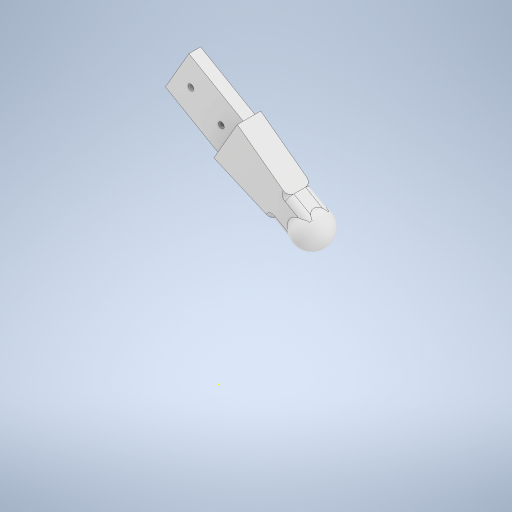
# Autodesk Inventor part: BR_parts_06(2)
Saved by Autodesk Inventor 2024.3 (Build 283343000, 343)
## iProperties
Created: 2024-10-20
Part Number: BR_parts_06(2)
Material: ABS プラスチック
Document SubType Name: Modeling
Designer: 佐藤智貴
Density: 1.06 g/cm^3
Appearance: 滑らか - 白
Mass: 50.0826 g
Surface Area: 111.12 cm^2
Volume: 47.2477 cm^3
Author: 佐藤智貴
Autodesk Inventor part; units mm, degrees
ref_plane "YZ Plane" through (0, 0, 0) normal (1, 0, 0) x (0, 1, 0)
ref_plane "XZ Plane" through (0, 0, 0) normal (0, 1, 0) x (-1, 0, 0)
ref_plane "XY Plane" through (0, 0, 0) normal (0, 0, 1) x (1, 0, 0)
sketch "スケッチ1" plane through (0, 0, 0) normal (0, 0, 1) x (1, 0, 0)
  line L0 (0, 0) -> (40, 0)
  line L1 (40, 0) -> (40, 318)
  line L2 (40, 318) -> (0, 318)
  line L3 (0, 318) -> (0, 0)
  line L4 (0, 218) -> (112.76268, 152.896436)
  line L5 (112.76268, 152.896436) -> (132.76268, 187.537452)
  line L6 (132.76268, 187.537452) -> (40, 241.094011)
  point P0 (40, 218)
  point P1 (40, 194.905989)
  point P2 (20, 318)
  point P3 (122.76268, 170.216944)
  point P4 (20, 258)
  dimension "d0" = 40
  dimension "d1" = 318
  dimension "d69" = 40
  dimension "d70" = 60
  dimension "d91" = 20
  dimension "d92" = 100
  dimension "d93" = 180
  dimension "d96" = 20
  dimension "d97" = 60
  constraints: 14 end point, 3 perpendicular, 3 point on line, 2 midpoint, 2 parallel, 1 horizontal
  measures "d0" distance of L1.end L2.end
  measures "d1" distance of L0.end L1.end
  measures "d69" distance of L4.end L5.end
  measures "d70" angle of L3 L4
  measures "d91" distance from line of L6 point (40, 218)
  measures "d92" distance from line of L2 L4.start
  measures "d93" distance of point (20, 318) point (122.763, 170.217)
  measures "d96" distance from line of L1 point (20, 258)
  measures "d97" distance from line of L2 point (20, 258)
extrude "押し出し1" add sketch "スケッチ1" along normal blind 19.6 contours L3 L2 L1 L4 | L1 L6 L5 L4
sketch "スケッチ6" plane through (0, 0, 19.6) normal (0, 0, 1) x (1, 0, 0)
  circle A0 centre (20, 258) radius 4
  line L0 (40, 318) -> (0, 318)
  line L1 (40, 241.094011) -> (40, 318)
  circle A1 centre (20, 20) radius 1.2295
  circle A2 centre (20, 10) radius 1.2295
  line L2 (0, 0) -> (40, 0)
  circle A3 centre (20, 298) radius 4
  point P0 (20, 318)
  point P1 (40, 190.811367)
  point P2 (30, 0)
  dimension "d42" = 8
  dimension "d44" = 20
  dimension "d45" = 2.459
  dimension "d46" = 2.459
  dimension "d47" = 10
  dimension "d48" = 10
  dimension "d49" = 20
  dimension "d50" = 20
  dimension "d53" = 8
  dimension "d54" = 20
  dimension "d55" = 40
  dimension "d56" = 20
  constraints: 4 centre point, 1 midpoint
  measures "d42" diameter of A0
  measures "d44" distance from line of L1 A0.centre
  measures "d45" diameter of A1
  measures "d46" diameter of A2
  measures "d47" distance from line of L2 A2.centre
  measures "d48" distance of A2.centre A1.centre
  measures "d49" distance from line of L1 A2.centre
  measures "d50" distance from line of L1 A1.centre
  measures "d53" diameter of A3
  measures "d54" distance from line of L0 A3.centre
  measures "d55" distance of A3.centre A0.centre
  measures "d56" distance from line of L1 A3.centre
extrude "押し出し4" cut sketch "スケッチ6" against normal through all
sketch "スケッチ8" plane through (0, 0, 0) normal (-1, 0, 0) x (0, 0, 1)
  line L0 (0, 318) -> (19.6, 318) projected
  line L1 (5, 318) -> (14.6, 318)
  line L2 (14.6, 318) -> (14.6, 278)
  line L3 (14.6, 278) -> (5, 278)
  line L4 (5, 278) -> (5, 318)
  line L5 (0, 318) -> (0, 0) projected
  dimension "d57" = 5
  dimension "d58" = 9.6
  dimension "d59" = 40
  dimension "d98" = 19.6
  constraints: 8 end point, 2 parallel, 1 horizontal, 1 perpendicular, 1 point on line
  measures "d57" distance between parallel lines of L5 L4
  measures "d58" distance between parallel lines of L4 L2
  measures "d59" distance between parallel lines of L0 L3
  measures "d98" distance of L0.start L0.end
extrude "押し出し5" cut sketch "スケッチ8" against normal through all
fillet "フィレット1" radius 20 4 edges at (40, 318, 17.1) (40, 318, 2.5) (0, 318, 2.5) (0, 318, 17.1)
fillet "フィレット2" radius 40 2 edges at (0, 218, 9.8) (40, 241.094, 9.8)
sketch "スケッチ9" plane through (0, 0, 19.6) normal (0, 0, 1) x (1, 0, 0)
  line L0 (20, 206.452995) -> (112.76268, 152.896436)
  line L1 (132.76268, 187.537452) -> (60, 229.547005)
  line L2 (112.76268, 152.896436) -> (132.76268, 187.537452)
  line L3 (132.76268, 187.537452) -> (112.76268, 152.896436)
  line L4 (66.38134, 179.674715) -> (112.76268, 152.896436)
  line L5 (132.76268, 187.537452) -> (166.773023, 167.901572)
  line L6 (115.120404, 126.980134) -> (133.517388, 158.844644)
  line L7 (141.753061, 173.109249) -> (128.76268, 180.609249)
  line L8 (112.76268, 152.896436) -> (20, 206.452995)
  line L9 (132.76268, 187.537452) -> (60, 229.547005)
  line L10 (115.120404, 126.980134) -> (125.753061, 145.396436)
  line L11 (133.517388, 158.844644) -> (145.753061, 180.037452)
  line L12 (116.76268, 159.824639) -> (129.753061, 152.324639)
  line L13 (66.38134, 179.674715) -> (129.753061, 152.324639)
  line L14 (66.38134, 179.674715) -> (86.38134, 214.315732)
  line L15 (86.38134, 214.315732) -> (141.753061, 173.109249)
  point P0 (0, 0)
  point P1 (254.453238, 80.328959)
  point P2 (128.76268, 180.609249)
  point P3 (123.257871, 156.074639)
  point P4 (86.38134, 214.315732)
  point P5 (40, 194.905989)
  point P6 (115.88749, 158.308766)
  point P7 (129.63787, 182.125122)
  dimension "d80" = 24
  dimension "d81" = 40
  dimension "d83" = 15
  dimension "d84" = 8
  dimension "d90" = 24
  constraints: 26 end point, 9 point on line, 6 perpendicular, 2 collinear, 2 midpoint, 1 parallel
  measures "d80" distance from line of point (254.453, 80.329) L7
  measures "d81" distance of L0.end L1.start
  measures "d83" distance between parallel lines of L2 L6
  measures "d84" distance between parallel lines of L5 L7
  measures "d90" distance from line of point (123.258, 156.075) L7
extrude "押し出し6" cut sketch "スケッチ9" against normal through all contours L13 L2 L0 | L1 L2 L15
sketch "スケッチ11" plane through (104.989657, 139.433165, 24) normal (0.8660254, -0.5, 0) x (0, 0, -1)
  line L0 (4.4, 21.795667) -> (4.4, 49.296427)
  line L1 (24, 21.795667) -> (24, 49.296427)
  line L2 (0, 24) -> (24, 24)
  line L3 (24, 24) -> (24, 0)
  line L4 (24, 0) -> (0, 0)
  line L5 (0, 0) -> (0, 24)
  line L6 (17, 17) -> (7, 17)
  line L7 (7, 17) -> (7, 7)
  line L8 (7, 7) -> (17, 7)
  line L9 (17, 7) -> (17, 17)
  line L10 (4.4, 35.546047) -> (24, 35.546047)
  circle A0 centre (14.2, 35.546047) radius 5
  point P0 (24, -173.247491)
  point P1 (24, 24)
  point P2 (0, 15.546047)
  point P3 (24, 15.546047)
  dimension "d85" = 10
  dimension "d88" = 10
  constraints: 16 end point, 4 parallel, 2 perpendicular, 1 centre point, 1 horizontal, 1 midpoint, 4 other
  measures "d85" distance of L6.start L6.end
  measures "d88" diameter of A0
extrude "押し出し7" add sketch "スケッチ11" along normal blind 15 contours A0 L10 | L10 A0
fillet "フィレット4" radius 20 2 edges at (0, 278, 9.8) (40, 278, 9.8)
sketch "スケッチ12" plane through (0, 0, 19.6) normal (0, 0, 1) x (1, 0, 0)
  arc A0 (40, 264.188022) -> (60, 229.547005) centre (80, 264.188022) ccw
  line L0 (60, 229.547005) -> (40, 194.905989)
  line L1 (20, 206.452995) -> (66.38134, 179.674715)
  line L2 (40, 194.905989) -> (66.38134, 179.674715)
  arc A1 (40, 264.188022) -> (60, 229.547005) centre (80, 264.188022) ccw
  arc A2 (0, 241.094011) -> (20, 206.452995) centre (40, 241.094011) ccw
  arc A3 (0, 241.094011) -> (20, 206.452995) centre (40, 241.094011) ccw
  line L3 (20, 206.452995) -> (40, 194.905989)
  line L4 (40, 264.188022) -> (0, 264.188022)
  line L5 (0, 298) -> (0, 241.094011)
  line L6 (0, 241.094011) -> (0, 264.188022)
  line L7 (129.63787, 182.125122) -> (86.38134, 214.315732)
  line L8 (60, 229.547005) -> (86.38134, 214.315732)
  line L9 (86.38134, 214.315732) -> (129.63787, 182.125122)
  line L10 (115.88749, 158.308766) -> (129.63787, 182.125122)
  line L11 (125.26268, 174.547071) -> (120.26268, 165.886817)
  line L12 (66.38134, 179.674715) -> (115.88749, 158.308766)
  line L13 (115.88749, 158.308766) -> (66.38134, 179.674715)
  circle A4 centre (67.721086, 201.995223) radius 2.5
  circle A5 centre (41.740324, 216.995223) radius 2.5
  line L14 (60, 229.547005) -> (86.38134, 214.315732)
  line L15 (66.38134, 179.674715) -> (40, 194.905989)
  line L16 (86.38134, 214.315732) -> (66.38134, 179.674715)
  arc A6 (60, 229.547005) -> (40, 194.905989) centre (50, 212.226497) ccw
  line L17 (76.38134, 196.995223) -> (41.740324, 216.995223)
  circle A7 centre (12.29546, 233.995223) radius 1.5
  line L18 (40, 194.905989) -> (20, 206.452995)
  line L19 (20, 206.452995) -> (40, 241.094011)
  line L20 (40, 241.094011) -> (60, 229.547005)
  point P0 (0, 0)
  dimension "d99" = 20
  dimension "d100" = 20
  dimension "d101" = 5
  dimension "d102" = 5
  dimension "d105" = 10
  dimension "d110" = 30
  dimension "d111" = 3
  dimension "d112" = 30
  constraints: 32 end point, 6 centre point, 6 collinear, 6 point on circle, 5 tangent, 3 perpendicular, 3 point on line, 1 coincident, 1 horizontal, 1 midpoint, 1 parallel
  measures "d99" distance from line of L1 A4.centre
  measures "d100" distance from line of L1 L17.end
  measures "d101" diameter of A5
  measures "d102" diameter of A4
  measures "d105" distance of L17.start A4.centre
  measures "d110" distance of A4.centre L17.end
  measures "d111" diameter of A7
extrude "押し出し8" add sketch "スケッチ12" along normal blind 10 contours L8 L16 L17 A4 L0 | L0 A6 | A6 L1 L19 L20 | L17 A4 L16 L1 L0 | L7 L10 L12 L16
sketch "スケッチ13" plane through (0, 0, 0) normal (0, 0, -1) x (-1, 0, 0)
  line L0 (22.594749, 365.444201) -> (-163.044716, 365.444201)
  line L1 (-163.044716, 365.444201) -> (-163.044716, 69.867597)
  line L2 (-163.044716, 69.867597) -> (22.594749, 69.867597)
  line L3 (22.594749, 69.867597) -> (22.594749, 365.444201)
  point P0 (0, 0)
  constraints: 8 end point, 2 parallel, 1 horizontal, 1 perpendicular
extrude "押し出し9" cut sketch "スケッチ13" against normal blind 19.6
sketch "スケッチ14" plane through (0, 0, 29.6) normal (0, 0, 1) x (1, 0, 0)
  line L0 (66.38134, 179.674715) -> (115.88749, 158.308766)
  line L1 (86.38134, 214.315732) -> (60, 229.547005)
  line L2 (66.38134, 179.674715) -> (86.38134, 214.315732)
  line L3 (115.88749, 158.308766) -> (129.63787, 182.125122)
  line L4 (86.38134, 214.315732) -> (129.63787, 182.125122)
  line L5 (129.63787, 182.125122) -> (115.88749, 158.308766)
  line L6 (115.88749, 158.308766) -> (66.38134, 179.674715)
  point P0 (0, 0)
  constraints: 8 end point, 1 collinear, 1 perpendicular
extrude "押し出し10" add sketch "スケッチ14" along normal blind 5 and the other way blind 15
sketch "スケッチ16" plane through (129.63787, 182.125122, 34.6) normal (0.8660254, -0.5, 0) x (0, 0, -1)
  line L0 (20, 0) -> (0, 0)
  line L1 (8, 6.24962) -> (8, -33.75038)
  line L2 (0, 0) -> (8, 0)
  line L3 (8, 0) -> (8, -27.500759)
  line L4 (8, -27.500759) -> (0, -27.500759)
  line L5 (0, -27.500759) -> (0, 0)
  line L6 (20, -27.500759) -> (0, -27.500759)
  line L7 (20, 0) -> (8, 0)
  line L8 (8, 0) -> (8, -27.500759)
  line L9 (8, -27.500759) -> (20, -27.500759)
  line L10 (20, -27.500759) -> (20, 0)
  point P0 (34.6, -222.543918)
  point P1 (13, 0)
  point P2 (13, -27.500759)
  point P3 (20, -27.500759)
  dimension "d119" = 0
  constraints: 16 end point, 4 parallel, 2 horizontal, 2 perpendicular, 1 point on line
  measures "d119" distance between parallel lines of L6 L4
extrude "押し出し12" add sketch "スケッチ16" along normal blind 20
sketch "スケッチ18" plane through (146.958378, 172.125122, 34.6) normal (0.8660254, -0.5, 0) x (0, 0, -1)
  point P0 (34.6, -222.543918)
sketch "スケッチ20" plane through (146.958378, 172.125122, 34.6) normal (0.8660254, -0.5, 0) x (0, 0, -1)
  circle A0 centre (10, -13.75038) radius 15
  line L0 (0, 0) -> (0, -27.500759)
  line L1 (10, -13.75038) -> (10, 1.24962)
  line L2 (10, -13.75038) -> (10, -28.75038)
  point P0 (34.6, -222.543918)
  dimension "d123" = 30
  dimension "d124" = 10
  constraints: 4 end point, 2 point on circle, 1 centre point, 1 vertical
  measures "d123" diameter of A0
  measures "d124" distance from line of L0 L1.start
revolve "回転3" add sketch "スケッチ20" angle 360 about axis through (140.083188, 160.216944, 24.6) along (-0.5, -0.8660254, 0) contours A0 L2 L1
fillet "フィレット5" radius 5 4 edges at (124.5477, 153.3088, 34.6) (124.5477, 153.3088, 14.6) (138.2981, 177.1251, 34.6) (138.2981, 177.1251, 14.6)
equation "\"d45\" = d46"
equation "\"d48\" = d47"
equation "\"d50\" = d49"
equation "\"d101\" = d102"
